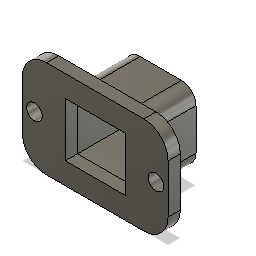
USB_B_Panel_Mount (Autodesk Fusion 360 design; units mm, degrees)
Autodesk Fusion 360 part; units mm, degrees
sketch "Sketch1" plane through (0, 0, 0) normal (0, 0, 1) x (1, 0, 0)
  line L0 (-4.25, 7.25) -> (4.25, 7.25)
  line L1 (7.25, 4.25) -> (7.25, -4.25)
  line L2 (4.25, -7.25) -> (-4.25, -7.25)
  line L3 (-7.25, -4.25) -> (-7.25, 4.25)
  line L4 (-7.25, 7.25) -> (7.25, -7.25) construction
  line L5 (7.25, 7.25) -> (-7.25, -7.25) construction
  arc A0 (-4.25, 7.25) -> (-7.25, 4.25) centre (-4.25, 4.25) ccw
  arc A1 (-7.25, -4.25) -> (-4.25, -7.25) centre (-4.25, -4.25) ccw
  arc A2 (4.25, -7.25) -> (7.25, -4.25) centre (4.25, -4.25) ccw
  arc A3 (7.25, 4.25) -> (4.25, 7.25) centre (4.25, 4.25) ccw
  line L6 (10, 10) -> (-10, 10)
  line L7 (-15, 5) -> (-15, -5)
  line L8 (-10, -10) -> (10, -10)
  line L9 (15, -5) -> (15, 5)
  line L10 (15, 10) -> (-15, -10) construction
  line L11 (-15, 10) -> (15, -10) construction
  arc A4 (15, 5) -> (10, 10) centre (10, 5) ccw
  arc A5 (-10, 10) -> (-15, 5) centre (-10, 5) ccw
  arc A6 (-15, -5) -> (-10, -10) centre (-10, -5) ccw
  arc A7 (10, -10) -> (15, -5) centre (10, -5) ccw
  circle A8 centre (-12.5, 0) radius 1.6
  line L12 (0, 0) -> (0, 5.6259) construction
  circle A9 centre (12.5, 0) radius 1.6
  line L13 (-3, 4.4279) -> (-3, -3.4951) construction
  line L14 (6.15, 5.55) -> (-6.15, 5.55)
  line L15 (-6.15, 5.55) -> (-6.15, -5.55)
  line L16 (-6.15, -5.55) -> (6.15, -5.55)
  line L17 (6.15, -5.55) -> (6.15, 5.55)
  line L18 (6.15, 5.55) -> (-6.15, -5.55) construction
  line L19 (-6.15, 5.55) -> (6.15, -5.55) construction
  line L20 (-6.35, -5.75) -> (6.35, -5.75)
  line L21 (6.35, -5.75) -> (6.35, 5.75)
  line L22 (6.35, 5.75) -> (-6.35, 5.75)
  line L23 (-6.35, 5.75) -> (-6.35, -5.75)
  dimension "d1" = 14.5
  dimension "d2" = 14.5
  dimension "d3" = 3
  dimension "d4" = 30
  dimension "d5" = 20
  dimension "d6" = 5
  dimension "d7" = 3.2
  dimension "d17" = 12.5
  dimension "d21" = 12.3
  dimension "d22" = 11.1
  dimension "d23" = 0.2
  constraint horizontal L0
  constraint perpendicular L0 L1
  constraint parallel L0 L2
  constraint parallel L1 L3
  constraint coincident L4.start L0
  constraint coincident L4.start L3
  constraint tangent L0 A0
  constraint tangent L3 A0
  constraint coincident L5.end L2
  constraint coincident L5.end L3
  constraint tangent L2 A1
  constraint tangent L3 A1
  constraint equal A0 A1
  constraint coincident L4.end L2
  constraint coincident L4.end L1
  constraint tangent L2 A2
  constraint tangent L1 A2
  constraint equal A0 A2
  constraint coincident L5.start L0
  constraint coincident L5.start L1
  constraint tangent L0 A3
  constraint tangent L1 A3
  constraint equal A0 A3
  constraint horizontal L6
  constraint perpendicular L6 L7
  constraint parallel L6 L8
  constraint parallel L7 L9
  constraint coincident L10.start L9
  constraint coincident L10.start L6
  constraint tangent L9 A4
  constraint tangent L6 A4
  constraint coincident L11.start L6
  constraint coincident L11.start L7
  constraint tangent L6 A5
  constraint tangent L7 A5
  constraint equal A4 A5
  constraint coincident L10.end L8
  constraint coincident L10.end L7
  constraint tangent L8 A6
  constraint tangent L7 A6
  constraint equal A4 A6
  constraint coincident L11.end L8
  constraint coincident L11.end L9
  constraint tangent L8 A7
  constraint tangent L9 A7
  constraint equal A4 A7
  constraint symmetric A8 L12 A9
  constraint horizontal L14
  constraint perpendicular L14 L15
  constraint parallel L14 L16
  constraint parallel L15 L17
  constraint coincident L18 L12.start
  constraint coincident L19 L12.start
  constraint coincident L12.start origin
  measures "d1" distance of L4.end L5.end
  measures "d2" distance of L5.start L4.end
  measures "d3" radius of A0
  measures "d4" distance of L10.end L11.end
  measures "d5" distance of L11.start L10.end
  measures "d6" radius of A4
  measures "d7" diameter of A8
  measures "d17" distance of L12.start A8.centre
  measures "d21" distance of L15.end L16.end
  measures "d22" distance of L14.end L15.end
extrude "Extrude1" add sketch "Sketch1" along normal blind 2.5 contours L0 L1 L2 L3 A0 A1 A2 A3 | L6 L7 L8 L9 A4 A5 A6 A7 | L20 L21 L22 L23
extrude "Extrude2" add sketch "Sketch1" against normal blind 11 contours L0 L1 L2 L3 A0 A1 A2 A3
